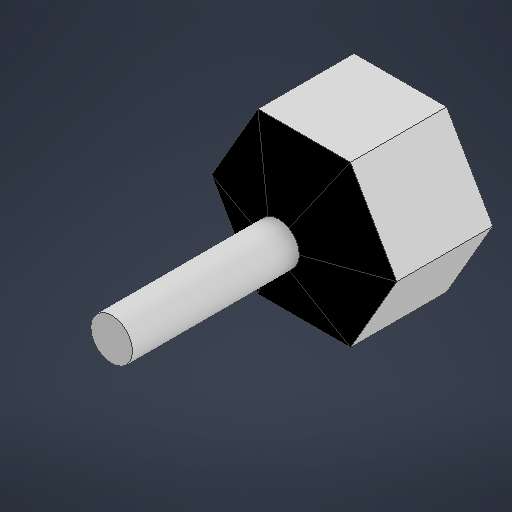
# Autodesk Inventor part: FeedThroughCap
Saved by Autodesk Inventor 2026.2 (Build 302298010, 298A)
## iProperties
Created: 2026-06-22
Part Number: FeedThroughCap
Material: Generic
Document SubType Name: Modeling
Designer: sonata
Density: 1 g/cm^3
Appearance: Default
Author: sonata
Autodesk Inventor part; units mm, degrees
ref_plane "YZ Plane" through (0, 0, 0) normal (1, 0, 0) x (0, 1, 0)
ref_plane "XZ Plane" through (0, 0, 0) normal (0, 1, 0) x (-1, 0, 0)
ref_plane "XY Plane" through (0, 0, 0) normal (0, 0, 1) x (1, 0, 0)
sketch "Sketch1" plane through (0, 0, 0) normal (0, 0, 1) x (1, 0, 0)
  line L0 (-1.8331, 0) -> (-0.9165, 1.5875)
  line L1 (-0.9165, 1.5875) -> (0.9165, 1.5875)
  line L2 (0.9165, 1.5875) -> (1.8331, 0)
  line L3 (1.8331, 0) -> (0.9165, -1.5875)
  line L4 (0.9165, -1.5875) -> (-0.9165, -1.5875)
  line L5 (-0.9165, -1.5875) -> (-1.8331, 0)
  line L6 (0, -1.5875) -> (0, 1.5875) construction
  point P0 (0, 0)
  dimension "d1" = 0
  dimension "d3" = 120
  dimension "d7" = 3.175
  constraints: 14 end point, 5 equal length, 2 horizontal alignment, 2 midpoint, 1 horizontal, 1 parallel
  measures "d1" distance from line of point (0, 0) L6
  measures "d3" angle of L3 L2
  measures "d7" distance between parallel lines of L1 L4
extrude "Extrusion1" add sketch "Sketch1" along normal blind 1.905
sketch "Sketch2" plane through (0, 0, 1.905) normal (0, 0, 1) x (1, 0, 0)
  circle A0 centre (0, 0) radius 0.4128
  dimension "d6" = 0.8255
  constraints: 1 centre point, 1 coincident
  measures "d6" diameter of A0
extrude "Extrusion2" add sketch "Sketch2" along normal blind 0.508
loft "Loft1" add section 1 edges at (-0.4128, 0, 2.413) section 2 edges at (0, -1.5875, 1.905) (1.3748, -0.7937, 1.905) (1.3748, 0.7938, 1.905) (0, 1.5875, 1.905) (-1.3748, 0.7937, 1.905) (-1.3748, -0.7938, 1.905)
sketch "Sketch3" plane through (0, 0, 2.413) normal (0, 0, 1) x (1, 0, 0)
  arc A0 (-0.2064, 0.3575) -> (-0.4128, 0) centre (0, 0) ccw projected
  circle A1 centre (0, 0) radius 0.4128
  arc A2 (0.4128, 0) -> (0.2064, 0.3575) centre (0, 0) ccw projected
  point P0 (0.3575, 0.2064)
  point P1 (-0.4128, 0)
  dimension "d15" = 0.8255
  constraints: 1 centre point, 1 coincident, 1 point on circle
  measures "d15" diameter of A1
extrude "Extrusion3" add sketch "Sketch3" along normal blind 3.302
body "Solid1"
